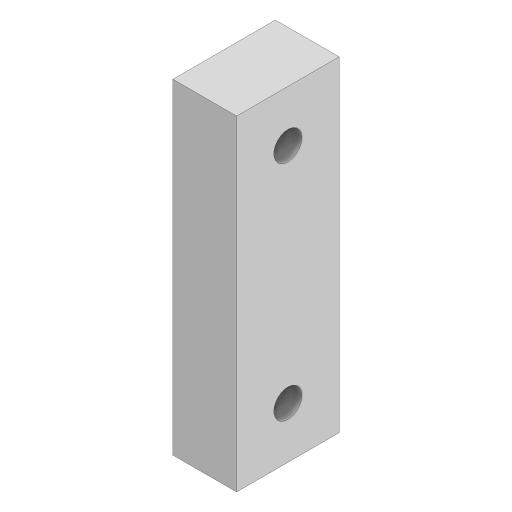
# Autodesk Inventor part: TOPE_CHUMACERA
Saved by Autodesk Inventor 2024 (Build 280153000, 153)
## iProperties
Created: 2024-08-28
Part Number: TOPE_CHUMACERA
Material: Generic
Document SubType Name: Modeling
Designer: Jhuliams
Density: 1 g/cm^3
Appearance: Default
Author: Jhuliams
Autodesk Inventor part; units mm, degrees
ref_plane "YZ Plane" through (0, 0, 0) normal (1, 0, 0) x (0, 1, 0)
ref_plane "XZ Plane" through (0, 0, 0) normal (0, 1, 0) x (-1, 0, 0)
ref_plane "XY Plane" through (0, 0, 0) normal (0, 0, 1) x (1, 0, 0)
sketch "Sketch1" plane through (0, 0, 0) normal (1, 0, 0) x (0, 1, 0)
  line L0 (27.65, 6.65) -> (-27.65, 6.65)
  line L1 (-27.65, 6.65) -> (-27.65, -6.65)
  line L2 (-27.65, -6.65) -> (27.65, -6.65)
  line L3 (27.65, -6.65) -> (27.65, 6.65)
  line L4 (27.65, 6.65) -> (-27.65, -6.65) construction
  line L5 (-27.65, 6.65) -> (27.65, -6.65) construction
  line L6 (30.65, -9.65) -> (-30.65, -9.65)
  line L7 (-30.65, -9.65) -> (-30.65, 9.65)
  line L8 (-30.65, 9.65) -> (30.65, 9.65)
  line L9 (30.65, 9.65) -> (30.65, -9.65)
  point P0 (0, 0)
  dimension "d0" = 55.3
  dimension "d1" = 13.3
  dimension "d2" = 3
  constraints: 20 end point, 4 parallel, 2 midpoint, 2 perpendicular, 1 horizontal, 3 other
  measures "d0" distance of L2.end L1.end
  measures "d1" distance of L1.end L0.end
  measures "d2" distance between parallel lines of L2 L6
extrude "Extrusion1" add sketch "Sketch1" along normal blind 12
sketch "Sketch2" plane through (12, 0, 0) normal (1, 0, 0) x (0, 0, -1)
  line L0 (-9.65, 30.65) -> (-9.65, -30.65) projected
  line L1 (-9.65, -30.65) -> (9.65, -30.65) projected
  line L2 (9.65, -30.65) -> (9.65, 30.65) projected
  line L3 (9.65, 30.65) -> (-9.65, 30.65) projected
  line L4 (-6.65, 27.65) -> (6.65, 27.65) projected
  line L5 (6.65, 27.65) -> (6.65, -27.65) projected
  line L6 (6.65, -27.65) -> (-6.65, -27.65) projected
  line L7 (-6.65, -27.65) -> (-6.65, 27.65) projected
  point P0 (0, 0)
extrude "Extrusion2" add sketch "Sketch2" against normal blind 11.5 contours L3 L2 L1 L0 | L4 L5 L6 L7
sketch "Sketch3" plane through (12, 0, 0) normal (1, 0, 0) x (0, 0, -1)
  line L0 (0, 0) -> (0, 21)
  line L1 (0, 0) -> (5, 0)
  circle A0 centre (0, 21) radius 2.65
  circle A1 centre (0, -21) radius 2.65
  dimension "d7" = 21
  dimension "d8" = 5
  dimension "d9" = 5.3
  constraints: 4 end point, 2 centre point, 1 coincident, 1 horizontal, 1 symmetric about line, 1 vertical, 1 other
  measures "d7" distance of L0.start L0.end
  measures "d8" distance of L0.start L1.end
  measures "d9" diameter of A0
extrude "Extrusion3" cut sketch "Sketch3" against normal blind 13
body "Solid1"
